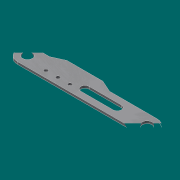
# Autodesk Inventor part: rinnku
Saved by Autodesk Inventor 2016 (Build 200138000, 138)
## iProperties
Created: 2016-08-23
Part Number: rinnku
Material: GFRP
Document SubType Name: Modeling
Designer: hiro
Density: 1.75 g/cm^3
Appearance: 滑らか - 淡い灰色
Mass: 6.14531 g
Surface Area: 43.3352 cm^2
Volume: 3.5116 cm^3
Author: hiro
Autodesk Inventor part; units mm, degrees
ref_plane "YZ Plane" through (0, 0, 0) normal (1, 0, 0) x (0, 1, 0)
ref_plane "XZ Plane" through (0, 0, 0) normal (0, 1, 0) x (-1, 0, 0)
ref_plane "XY Plane" through (0, 0, 0) normal (0, 0, 1) x (1, 0, 0)
sketch "スケッチ1" plane through (0, 0, 0) normal (0, 0, 1) x (1, 0, 0)
  line L0 (-50, 0) -> (50, 0) construction
  circle A0 centre (-50, 0) radius 4.05
  circle A1 centre (50, 0) radius 4.05
  line L1 (-50, 8.5) -> (43, 8.5)
  line L2 (-50, -8.5) -> (43, -8.5)
  arc A2 (-50, 8.5) -> (-50, -8.5) centre (-50, 0) ccw
  arc A3 (25.013, -3.45) -> (25.013, 3.45) centre (25.013, 0) ccw
  line L3 (25.013, -3.45) -> (-2, -3.45)
  line L4 (25.013, 3.45) -> (-2, 3.45)
  arc A4 (-2, 3.45) -> (-2, -3.45) centre (-2, 0) ccw
  line L5 (43, -8.5) -> (50.0601, -8.4498)
  line L6 (43, 8.5) -> (50.0601, 8.4498)
  arc A5 (50.0601, -8.4498) -> (50.0601, 8.4498) centre (50, 0) ccw
  line L7 (0, 13) -> (-30, 13)
  line L8 (-30, 13) -> (-40, 8.5)
  line L9 (0, 13) -> (10, 8.5)
  circle A6 centre (-2, 0) radius 7 construction
  line L10 (-26.5125, -1.6815) -> (-20.6511, -11.8338) construction
  line L11 (-20.6511, -11.8338) -> (-53.7549, -30.9463) construction
  line L12 (-53.7549, -30.9463) -> (-59.6163, -20.794) construction
  line L13 (-59.6163, -20.794) -> (-26.5125, -1.6815) construction
  line L14 (-13.6037, 7.7659) -> (-48.3091, -4.7054) construction
  arc A7 (-13.6037, 7.7659) -> (-27.0705, 29.3127) centre (-18, 20) ccw construction
  line L15 (-27.0705, 29.3127) -> (-53.4886, 3.5818) construction
  arc A8 (-53.4886, 3.5818) -> (-48.3091, -4.7054) centre (-50, 0) ccw construction
  circle A9 centre (-10.3371, -5.2455) radius 1.55
  circle A10 centre (-17.0592, -2.5296) radius 1.55
  circle A11 centre (-23.7813, 0.1863) radius 1.55
  line L16 (-10.3371, -5.2455) -> (-23.7813, 0.1863) construction
  circle A12 centre (-10.3371, -5.2455) radius 2.85 construction
  line L17 (-8.9556, -8.5) -> (-7.0826, -3.8641) construction
  line L18 (-7.0826, -3.8641) -> (-25.1627, 3.4407) construction
  line L19 (-25.1627, 3.4407) -> (-27.0357, -1.1952) construction
  line L20 (-27.0357, -1.1952) -> (-8.9556, -8.5) construction
  line L21 (-10.3371, -5.2455) -> (-8.0191, -6.182) construction
  line L22 (-17.0592, -2.5296) -> (-17.9957, -4.8476) construction
  line L23 (-26.5125, -1.6815) -> (-28.0429, 2.5772) construction
  line L24 (-24.2542, -2.319) -> (-11.7372, -7.3762) construction
  line L25 (-11.7372, -7.3762) -> (-10.8007, -5.0582) construction
  line L26 (-10.8007, -5.0582) -> (-23.3177, -0.001) construction
  line L27 (-23.3177, -0.001) -> (-24.2542, -2.319) construction
  circle A13 centre (-17.0592, -2.5296) radius 2.85 construction
  point P0 (0, 0)
  point P1 (0, 0)
  dimension "d0" = 100
  dimension "d1" = 8.1
  dimension "d2" = 8.5
  dimension "d5" = 3.45
  dimension "d7" = 52
  dimension "d8" = 8.1
  dimension "d9" = 7
  dimension "d10" = 8.45
  dimension "d11" = 27.013
  dimension "d17" = 13
  dimension "d19" = 10
  dimension "d20" = 30
  dimension "d22" = 10
  dimension "d23" = 40
  dimension "d29" = 14
  dimension "d32" = 19.5
  dimension "d33" = 13.2
  dimension "d34" = 5
  dimension "d35" = 20
  dimension "d36" = 32
  dimension "d37" = 13
  dimension "d38" = 120
  dimension "d40" = 3.1
  dimension "d41" = 5.7
  dimension "d42" = 14.5
  dimension "d43" = 5
  dimension "d44" = 2.5
  dimension "d49" = 3
  dimension "d50" = 22
  constraints: 56 end point, 14 centre point, 13 tangent, 12 point on circle, 10 perpendicular, 9 coincident, 6 point on line, 5 horizontal, 4 midpoint, 3 equal radius, 3 parallel, 2 horizontal alignment, 1 vertical alignment, 1 other
  measures "d0" distance of L0.start L0.end
  measures "d1" diameter of A0
  measures "d2" radius of A2
  measures "d5" radius of A3
  measures "d7" distance of L0.end A4.centre
  measures "d8" diameter of A1
  measures "d9" horizontal distance of L1.end L0.end
  measures "d10" radius of A5
  measures "d11" distance of A4.centre A3.centre
  measures "d17" distance from line of L0.end L7
  measures "d19" horizontal distance of L8.end L7.end
  measures "d20" distance of L7.start L7.end
  measures "d22" horizontal distance of L9.end L7.start
  measures "d23" horizontal distance of L0.end L9.end
  measures "d29" diameter of A6
  measures "d32" distance from line of L0.start L10
  measures "d33" distance from line of L0.start L13
  measures "d34" radius of A8
  measures "d35" vertical distance of L0.start A7.centre
  measures "d36" horizontal distance of L0.start A7.centre
  measures "d37" radius of A7
  measures "d38" angle of L2 L10
  measures "d40" diameter of A9
  measures "d41" diameter of A12
  measures "d42" distance of L16.start L16.end
  measures "d43" distance of L17.start L17.end
  measures "d44" distance from line of L17 L21.start
  measures "d49" distance between parallel lines of L19 L27
  measures "d50" angle of L2 L24
extrude "押し出し1" add sketch "スケッチ1" along normal blind 2
fillet "フィレット1" radius 2 4 edges at (-40, 8.5, 1) (-30, 13, 1) (0, 13, 1) (43, 8.5, 1)
equation "\"d7\" = 2 * d28"
equation "\"d8\" = d1"
equation "\"d11\" = d39"
equation "\"d19\" = d18"
equation "\"d22\" = d19"
equation "\"d28\" = 26"
equation "\"d39\" = 27.012989"
equation "\"d18\" = 10"
